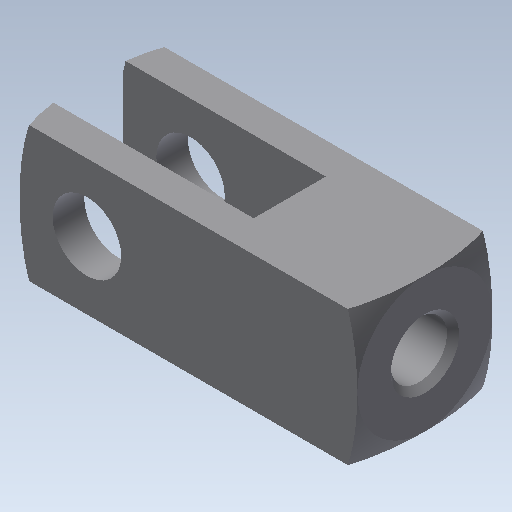
# Autodesk Inventor part: D-14043
Saved by Autodesk Inventor 2020 (Build 240168000, 168)
## iProperties
Created: 2020-01-07
Part Number: D-14043
Material: Generic
Catalog Web Link: www.cadenas.de
Description: Piston Rod Clevis for Original Line Cylinders - Body-
Vendor: BIMBA
Document SubType Name: Modeling
Designer: psadmin
Manufacturer: BIMBA
Mass: 1.26173 g
Surface Area: 12.864 cm^2
Volume: 1.26173 cm^3
Density: 1 g/cm^3
Appearance: PSOLRGB-191-191-191
Category: PARTsolutions
Company: BIMBA
PSOL_IDENT_0: {$CADENAS_DATA\23d-libs\bimba\bimba_brand\bimba_imperial\bimba_full_line\original_line_cylinders\acc
PSOL_IDENT_1: essories\piston_rod_clevis_body.prj},201 {VTYP=3D},{NB=D-14043},{LINA=D-14043},{NN=Piston Rod Clevis
PSOL_IDENT_2: for Original Line Cylinders - Body},{DATE=23.12.2019 10:36:51},{GEOMDATE=06.12.2012 07:16:06},{VERS
PSOL_IDENT_3: ION=},{LINEID=190},{WBVAR=},{WBNUMERIC=}  {NB=D-14043},{LINA=D-14043},{KT=DUMMY},{PN=D-14043},{L=0.9
PSOL_IDENT_4: 3700000},{L1=0.75000000},{L2=0.37500000},{W=0.20000000},{W1=0.37500000},{DIA1=0.19000000},{DIA1CS=0.
PSOL_IDENT_5: 00000000},{DIA2=0.37500000},{DIA3=0.15620000},{CS=90.00000000},{CDP=0.03000000},{AN=30.00000000},{ND
PSOL_IDENT_6: M=0.19000000},{CODE=UNF},{NDMDP=0.31000000},{COLOR=0.75,0.75,0.75,0.00}
NN: Piston Rod Clevis for Original Line Cylinders - Body
NB: D-14043
NBSYN: $PN.
LINA: D-14043
PN: D-14043
L: 0.937
L1: 0.75
L2: 0.375
W: 0.2
W1: 0.375
DIA1: 0.19
DIA1CS: 0
DIA2: 0.375
DIA3: 0.1562
CS: 90
CDP: 0.03
AN: 30
NDM: 0.19
CODE: UNF
NDMDP: 0.31
SUPPLIER: BIMBA
ARTICLENO: D-14043
BOMINFO: D-14043
CREATOR: CADENAS GmbH
d21: 0.000 in
d22: 0.000 in
Title: D-14043
Author: Cadenas PARTsolutions
Autodesk Inventor part; units mm, degrees
sketch "Sketch_1" plane through (0, 0, 0) normal (0, 0, 1) x (1, 0, 0)
  line L0 (-4.7498, -4.7625) -> (19.05, -4.7625)
  line L1 (19.05, -4.7625) -> (19.05, 4.7625)
  line L2 (19.05, 4.7625) -> (-4.7498, 4.7625)
  line L3 (-4.7498, 4.7625) -> (-4.7498, -4.7625)
  constraints: 8 end point
extrude "Extrusion1" add sketch "Sketch_1" along normal mid plane 9.525
sketch "Sketch_2" plane through (0, 0, 0) normal (0, 1, 0) x (-1, 0, 0)
  line L0 (4.7498, 2.54) -> (-9.525, 2.54)
  line L1 (-9.525, 2.54) -> (-9.525, -2.54)
  line L2 (-9.525, -2.54) -> (4.7498, -2.54)
  line L3 (4.7498, -2.54) -> (4.7498, 2.54)
  constraints: 8 end point
extrude "Extrusion2" cut sketch "Sketch_2" along normal mid plane 9.525
sketch "Sketch_3" plane through (0, 0, 0) normal (0, 0, 1) x (1, 0, 0)
  line L0 (19.05, 0) -> (11.176, 0)
  line L1 (11.176, 0) -> (11.176, 1.9837)
  line L2 (11.176, 1.9837) -> (18.6207, 1.9837)
  line L3 (18.6207, 1.9837) -> (19.05, 2.413)
  line L4 (19.05, 2.413) -> (19.05, 0)
  line L5 (19.05, 0) -> (11.176, 0)
  constraints: 12 end point
revolve "Revolution1" cut sketch "Sketch_3" angle 360 about axis through (19.05, 0, 0) along (1, 0, 0)
sketch "Sketch5" plane through (11.176, 0, 0) normal (1, 0, 0) x (0, 0, -1)
  point P0 (0, 0)
hole "Hole1" at (11.176, 0, 0) direction (-1, 0, 0) diameter 3.9675 depth 1.651
sketch "Sketch6" plane through (0, 0, -4.7625) normal (0, 0, -1) x (-1, 0, 0)
  point P0 (0, 0)
hole "Hole2" at (0, 0, -4.7625) direction (0, 0, 1) diameter 4.826 depth 9.525
sketch "Sketch_9" plane through (0, 0, 0) normal (0, 0, 1) x (1, 0, 0)
  line L0 (23.8125, 0) -> (19.05, 0)
  line L1 (19.05, 0) -> (19.05, 4.7625)
  arc A0 (19.05, 4.7625) -> (16.51, 9.525) centre (8.8503, 2.3812) ccw
  line L2 (16.51, 9.525) -> (23.8125, 9.525)
  line L3 (23.8125, 9.525) -> (23.8125, 0)
  line L4 (23.8125, 0) -> (19.05, 0)
  constraints: 10 end point, 2 point on circle, 1 centre point
revolve "Revolution2" cut sketch "Sketch_9" angle 360 about axis through (23.8125, 0, 0) along (1, 0, 0)
sketch "Sketch_10" plane through (0, 0, 0) normal (0, 0, 1) x (1, 0, 0)
  line L0 (-4.7498, 0) -> (-9.5123, 0)
  line L1 (-9.5123, 0) -> (-9.5123, 9.525)
  line L2 (-9.5123, 9.525) -> (-2.2098, 9.525)
  arc A0 (-2.2098, 9.525) -> (-4.7498, 4.7625) centre (5.4499, 2.3813) ccw
  line L3 (-4.7498, 4.7625) -> (-4.7498, 0)
  line L4 (-4.7498, 0) -> (-9.5123, 0)
  constraints: 10 end point, 2 point on circle, 1 centre point
revolve "Revolution3" cut sketch "Sketch_10" angle 360 about axis through (-4.7498, 0, 0) along (1, 0, 0)
ref_plane "dummy_XY" through (0, 0, 0) normal (0, 0, 1) x (1, 0, 0)
ref_plane "dummy_YZ" through (0, 0, 0) normal (1, 0, 0) x (0, 1, 0)
ref_plane "dummy_ZX" through (0, 0, 0) normal (0, 1, 0) x (0, 0, 1)
ref_plane "h1_XY" through (-4.7498, 4.7625, 0) normal (0, 0, 1) x (1, 0, 0)
ref_plane "h1_YZ" through (-4.7498, 4.7625, 0) normal (1, 0, 0) x (0, 1, 0)
ref_plane "h1_ZX" through (-4.7498, 4.7625, 0) normal (0, 1, 0) x (0, 0, 1)
ref_plane "h2_XY" through (-4.7498, -4.7625, 0) normal (0, 0, 1) x (1, 0, 0)
ref_plane "h2_YZ" through (-4.7498, -4.7625, 0) normal (1, 0, 0) x (0, 1, 0)
ref_plane "h2_ZX" through (-4.7498, -4.7625, 0) normal (0, 1, 0) x (0, 0, 1)
ref_plane "l1_XY" through (19.05, 4.7625, 0) normal (0, 0, 1) x (1, 0, 0)
ref_plane "l1_YZ" through (19.05, 4.7625, 0) normal (1, 0, 0) x (0, 1, 0)
ref_plane "l1_ZX" through (19.05, 4.7625, 0) normal (0, 1, 0) x (0, 0, 1)
ref_plane "l11_XY" through (19.05, 4.7625, 0) normal (0, 0, 1) x (1, 0, 0)
ref_plane "l11_YZ" through (19.05, 4.7625, 0) normal (1, 0, 0) x (0, 1, 0)
ref_plane "l11_ZX" through (19.05, 4.7625, 0) normal (0, 1, 0) x (0, 0, 1)
ref_plane "l12_XY" through (0, 4.7625, 0) normal (0, 0, 1) x (1, 0, 0)
ref_plane "l12_YZ" through (0, 4.7625, 0) normal (1, 0, 0) x (0, 1, 0)
ref_plane "l12_ZX" through (0, 4.7625, 0) normal (0, 1, 0) x (0, 0, 1)
ref_plane "l2_XY" through (-4.7498, 4.7625, 0) normal (0, 0, 1) x (1, 0, 0)
ref_plane "l2_YZ" through (-4.7498, 4.7625, 0) normal (1, 0, 0) x (0, 1, 0)
ref_plane "l2_ZX" through (-4.7498, 4.7625, 0) normal (0, 1, 0) x (0, 0, 1)
ref_plane "l21_XY" through (19.05, 0, 0) normal (0, 1, 0) x (1, 0, 0)
ref_plane "l21_YZ" through (19.05, 0, 0) normal (1, 0, 0) x (0, 0, -1)
ref_plane "l21_ZX" through (19.05, 0, 0) normal (0, 0, -1) x (0, 1, 0)
ref_plane "l22_XY" through (9.525, 0, 0) normal (0, 1, 0) x (1, 0, 0)
ref_plane "l22_YZ" through (9.525, 0, 0) normal (1, 0, 0) x (0, 0, -1)
ref_plane "l22_ZX" through (9.525, 0, 0) normal (0, 0, -1) x (0, 1, 0)
ref_plane "piston_rod_clevis_XY" through (19.05, 0, 0) normal (1, 0, 0) x (0, 0, -1)
ref_plane "piston_rod_clevis_YZ" through (19.05, 0, 0) normal (0, 0, -1) x (0, 1, 0)
ref_plane "piston_rod_clevis_ZX" through (19.05, 0, 0) normal (0, 1, 0) x (1, 0, 0)
ref_plane "rod_clevis_body_XY" through (0, 0, 0) normal (0, 0, 1) x (1, 0, 0)
ref_plane "rod_clevis_body_YZ" through (0, 0, 0) normal (1, 0, 0) x (0, 1, 0)
ref_plane "rod_clevis_body_ZX" through (0, 0, 0) normal (0, 1, 0) x (0, 0, 1)
ref_plane "th1_XY" through (19.05, 2.413, 0) normal (0, 0, 1) x (1, 0, 0)
ref_plane "th1_YZ" through (19.05, 2.413, 0) normal (1, 0, 0) x (0, 1, 0)
ref_plane "th1_ZX" through (19.05, 2.413, 0) normal (0, 1, 0) x (0, 0, 1)
ref_plane "th2_XY" through (19.05, -2.413, 0) normal (0, 0, 1) x (1, 0, 0)
ref_plane "th2_YZ" through (19.05, -2.413, 0) normal (1, 0, 0) x (0, 1, 0)
ref_plane "th2_ZX" through (19.05, -2.413, 0) normal (0, 1, 0) x (0, 0, 1)
ref_plane "to_cylinder_XY" through (9.525, 0, 0) normal (1, 0, 0) x (0, 0, -1)
ref_plane "to_cylinder_YZ" through (9.525, 0, 0) normal (0, 0, -1) x (0, 1, 0)
ref_plane "to_cylinder_ZX" through (9.525, 0, 0) normal (0, 1, 0) x (1, 0, 0)
ref_plane "w1_XY" through (19.05, 0, -4.7625) normal (0, 1, 0) x (1, 0, 0)
ref_plane "w1_YZ" through (19.05, 0, -4.7625) normal (1, 0, 0) x (0, 0, -1)
ref_plane "w1_ZX" through (19.05, 0, -4.7625) normal (0, 0, -1) x (0, 1, 0)
ref_plane "w11_XY" through (-4.7498, 0, -2.54) normal (0, 1, 0) x (1, 0, 0)
ref_plane "w11_YZ" through (-4.7498, 0, -2.54) normal (1, 0, 0) x (0, 0, -1)
ref_plane "w11_ZX" through (-4.7498, 0, -2.54) normal (0, 0, -1) x (0, 1, 0)
ref_plane "w12_XY" through (-4.7498, 0, 2.54) normal (0, 1, 0) x (1, 0, 0)
ref_plane "w12_YZ" through (-4.7498, 0, 2.54) normal (1, 0, 0) x (0, 0, -1)
ref_plane "w12_ZX" through (-4.7498, 0, 2.54) normal (0, 0, -1) x (0, 1, 0)
ref_plane "w2_XY" through (19.05, 0, 4.7625) normal (0, 1, 0) x (1, 0, 0)
ref_plane "w2_YZ" through (19.05, 0, 4.7625) normal (1, 0, 0) x (0, 0, -1)
ref_plane "w2_ZX" through (19.05, 0, 4.7625) normal (0, 0, -1) x (0, 1, 0)
body "Solid1"
